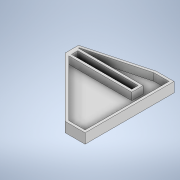
# Autodesk Inventor part: Speaker Stand
Saved by Autodesk Inventor 2021 (Build 250183000, 183)
## iProperties
Created: 2023-05-10
Part Number: Speaker Stand
Material: Generic
Document SubType Name: Modeling
Designer: mathe
Density: 1 g/cm^3
Appearance: Default
Author: mathe
Autodesk Inventor part; units mm, degrees
ref_plane "YZ Plane" through (0, 0, 0) normal (1, 0, 0) x (0, 1, 0)
ref_plane "XZ Plane" through (0, 0, 0) normal (0, 1, 0) x (-1, 0, 0)
ref_plane "XY Plane" through (0, 0, 0) normal (0, 0, 1) x (1, 0, 0)
sketch "Sketch1" plane through (0, 0, 0) normal (0, 1, 0) x (-1, 0, 0)
  line L0 (0, 0) -> (90, 0)
  line L1 (90, 0) -> (90, -90)
  line L2 (90, -90) -> (0, -90)
  line L3 (0, -90) -> (0, 0)
  line L4 (0, 0) -> (90, 0)
  line L5 (90, 0) -> (90, -65)
  line L6 (90, -65) -> (0, -65)
  line L7 (0, -65) -> (0, 0)
  line L8 (14.5, -68.2385) -> (75.5, -68.2385)
  line L9 (75.5, -68.2385) -> (75.5, -61.7615)
  line L10 (75.5, -61.7615) -> (14.5, -61.7615)
  line L11 (14.5, -61.7615) -> (14.5, -68.2385)
  line L12 (14.5, -68.2385) -> (75.5, -61.7615) construction
  line L13 (75.5, -68.2385) -> (14.5, -61.7615) construction
  line L14 (14.5, -68.2385) -> (75.5, -68.2385) construction
  point P0 (45, -65)
  dimension "d16" = 90
  dimension "d17" = 90
  dimension "d18" = 90
  dimension "d19" = 65
  dimension "d20" = 61
  dimension "d21" = 0
  dimension "d22" = 6.477
  constraints: 30 end point, 7 parallel, 3 horizontal, 3 midpoint, 3 perpendicular, 1 collinear
  measures "d16" distance of L1.end L2.end
  measures "d17" distance of L0.end L1.end
  measures "d18" distance of L5.end L6.end
  measures "d19" distance of L4.end L5.end
  measures "d20" distance of L8.start L8.end
  measures "d21" distance between parallel lines of L8 L14
  measures "d22" distance of L9.end L8.end
extrude "Extrusion1" add sketch "Sketch1" along normal blind 10 contours L0 L1 L6 L9 L10 L11 L3 | L6 L11 L8 L9 L1 L2 L3
chamfer "Chamfer1" distance 69.85 angle 45 1 edges at (-90, 5, 0)
sketch "Sketch2" plane through (-90, 0, -69.85) normal (-1, 0, 0) x (0, 0, 1)
  line L0 (69.85, 10) -> (0, 10) projected
  line L1 (0, 10) -> (0, 0) projected
  line L2 (0, 0) -> (69.85, 0) projected
  line L3 (69.85, 0) -> (69.85, 10) projected
  line L4 (-20.15, 0) -> (0, 0) projected
  line L5 (0, 10) -> (0, 0) projected
  line L6 (-20.15, 10) -> (0, 10) projected
  line L7 (-7.8336, 10) -> (-20.15, 10) projected
  line L8 (-20.15, 10) -> (-20.15, 0) projected
  line L9 (-20.15, 0) -> (-7.8336, 0) projected
  line L10 (-7.8336, 0) -> (-7.8336, 10) projected
  line L11 (-20.15, 0) -> (-20.15, 10) projected
extrude "Extrusion2" cut sketch "Sketch2" against normal blind 10
chamfer "Chamfer3" distance 61.9125 angle 15 1 edges at (-80, 5, -90) measured on face at (-26.6667, 6.6667, -90)
shell "Shell1" thickness 2.54 removed faces 1 at (-36.7167, 10, -41.1743)
body "Solid1"
